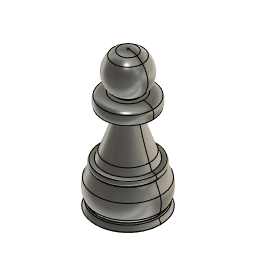
Pawn v1 (Autodesk Fusion 360 design; units mm, degrees)
Autodesk Fusion 360 part; units mm, degrees
sketch "pawn - side view" plane through (0, 0, 0) normal (0, 1, 0) x (1, 0, 0)
  spline S0 degree 3 poles (22.3033, -83.3947) (18.8902, -82.2834) (16.0063, -79.2936) (15.0802, -75.854) knots 0 0 0 0 1 1 1 1
  spline S1 degree 3 poles (15.0802, -75.854) (14.604, -74.0813) (14.7098, -71.1709) (15.3183, -69.3982) knots 0 0 0 0 1 1 1 1
  spline S2 degree 3 poles (15.3183, -69.3982) (15.9533, -67.5726) (16.5619, -66.6201) (18.361, -64.7944) knots 0 0 0 0 1 1 1 1
  line L0 (18.361, -64.7944) -> (19.684, -63.3922)
  line L1 (19.684, -63.3922) -> (17.1969, -63.3922)
  spline S3 degree 3 poles (17.1969, -63.3922) (15.239, -63.3922) (14.4981, -63.2863) (13.5985, -62.8365) knots 0 0 0 0 1 1 1 1
  spline S4 degree 3 poles (13.5985, -62.8365) (10.5558, -61.3813) (10.4235, -57.0686) (13.3604, -55.3753) knots 0 0 0 0 1 1 1 1
  spline S5 degree 3 poles (13.3604, -55.3753) (13.6515, -55.1901) (15.2125, -55.0049) (16.8, -54.9255) knots 0 0 0 0 1 1 1 1
  line L2 (16.8, -54.9255) -> (19.7104, -54.7932)
  line L3 (19.7104, -54.7932) -> (19.7898, -53.973)
  spline S6 degree 3 poles (19.7898, -53.973) (19.9485, -52.4384) (16.0592, -38.8124) (13.969, -33.5207) knots 0 0 0 0 1 1 1 1
  spline S7 degree 3 poles (13.969, -33.5207) (13.5456, -32.4359) (13.2546, -31.404) (13.334, -31.1924) knots 0 0 0 0 1 1 1 1
  spline S8 degree 3 poles (13.334, -31.1924) (13.5456, -30.6897) (38.3106, -30.6632) (38.5223, -31.1924) knots 0 0 0 0 1 1 1 1
  spline S9 degree 3 poles (38.5223, -31.1924) (38.6017, -31.404) (37.9667, -33.2032) (37.1465, -35.2405) knots 0 0 0 0 1 1 1 1
  spline S10 degree 3 poles (37.1465, -35.2405) (34.236, -42.3842) (30.8758, -53.3909) (31.2992, -54.4757) knots 0 0 0 0 1 1 1 1
  spline S11 degree 3 poles (31.2992, -54.4757) (31.4315, -54.8461) (31.8548, -54.9255) (34.0244, -54.9255) knots 0 0 0 0 1 1 1 1
  spline S12 degree 3 poles (34.0244, -54.9255) (36.9348, -54.9255) (38.0196, -55.2959) (38.9721, -56.6188) knots 0 0 0 0 1 1 1 1
  spline S13 degree 3 poles (38.9721, -56.6188) (39.7658, -57.7565) (39.7923, -60.3759) (38.9985, -61.4607) knots 0 0 0 0 1 1 1 1
  spline S14 degree 3 poles (38.9985, -61.4607) (38.0196, -62.8101) (36.4321, -63.3922) (33.8392, -63.3922) knots 0 0 0 0 1 1 1 1
  line L4 (33.8392, -63.3922) -> (31.5108, -63.3922)
  line L5 (31.5108, -63.3922) -> (32.966, -64.8474)
  spline S15 degree 3 poles (32.966, -64.8474) (37.3317, -69.213) (37.4904, -76.0392) (33.31, -80.4578) knots 0 0 0 0 1 1 1 1
  spline S16 degree 3 poles (33.31, -80.4578) (32.4104, -81.4103) (31.2992, -82.2305) (30.1879, -82.7597) knots 0 0 0 0 1 1 1 1
  spline S17 degree 3 poles (30.1879, -82.7597) (28.6533, -83.5005) (28.1242, -83.6063) (25.9281, -83.6857) knots 0 0 0 0 1 1 1 1
  spline S18 degree 3 poles (25.9281, -83.6857) (24.3142, -83.7386) (23.0177, -83.6328) (22.3033, -83.3947) knots 0 0 0 0 1 1 1 1
  spline S19 degree 3 poles (11.1115, -29.7901) (10.5294, -29.208) (10.3971, -27.6999) (10.8998, -27.1972) knots 0 0 0 0 1 1 1 1
  spline S20 degree 3 poles (10.8998, -27.1972) (11.1379, -26.959) (14.8156, -26.8797) (25.7958, -26.8797) knots 0 0 0 0 1 1 1 1
  spline S21 degree 3 poles (25.7958, -26.8797) (39.6071, -26.8797) (40.4273, -26.9061) (40.8242, -27.3559) knots 0 0 0 0 1 1 1 1
  spline S22 degree 3 poles (40.8242, -27.3559) (41.4856, -28.0967) (41.3798, -29.1286) (40.586, -29.7636) knots 0 0 0 0 1 1 1 1
  spline S23 degree 3 poles (40.586, -29.7636) (39.8981, -30.3192) (39.6335, -30.3192) (25.7694, -30.3192) knots 0 0 0 0 1 1 1 1
  spline S24 degree 3 poles (25.7694, -30.3192) (11.9846, -30.3192) (11.6406, -30.3192) (11.1115, -29.7901) knots 0 0 0 0 1 1 1 1
  spline S25 degree 3 poles (10.0267, -24.3132) (8.1746, -21.4028) (7.3015, -18.4924) (7.4867, -15.8201) knots 0 0 0 0 1 1 1 1
  spline S26 degree 3 poles (7.4867, -15.8201) (7.6454, -13.5182) (8.4921, -10.9517) (9.4181, -10.0257) knots 0 0 0 0 1 1 1 1
  line L6 (9.4181, -10.0257) -> (10.0267, -9.4172)
  line L7 (10.0267, -9.4172) -> (25.5313, -9.4172)
  spline S27 degree 3 poles (25.5313, -9.4172) (34.8181, -9.4172) (41.221, -9.523) (41.5121, -9.6817) knots 0 0 0 0 1 1 1 1
  spline S28 degree 3 poles (41.5121, -9.6817) (41.7767, -9.814) (42.3323, -10.6607) (42.7292, -11.5867) knots 0 0 0 0 1 1 1 1
  spline S29 degree 3 poles (42.7292, -11.5867) (43.814, -13.9415) (43.9727, -17.3017) (43.126, -20.0534) knots 0 0 0 0 1 1 1 1
  spline S30 degree 3 poles (43.126, -20.0534) (42.4381, -22.3024) (41.221, -24.8953) (40.4273, -25.7684) knots 0 0 0 0 1 1 1 1
  line L8 (40.4273, -25.7684) -> (39.8717, -26.3505)
  line L9 (39.8717, -26.3505) -> (25.6106, -26.3505)
  line L10 (25.6106, -26.3505) -> (11.3496, -26.3505)
  line L11 (11.3496, -26.3505) -> (10.0267, -24.3132)
  spline S31 degree 3 poles (8.8096, -8.4911) (8.1481, -8.0413) (7.7777, -6.6126) (8.0423, -5.5807) knots 0 0 0 0 1 1 1 1
  line L12 (8.0423, -5.5807) -> (8.201, -4.9192)
  line L13 (8.201, -4.9192) -> (25.3725, -4.9192)
  spline S32 degree 3 poles (25.3725, -4.9192) (40.639, -4.9192) (42.5969, -4.9722) (42.9673, -5.3426) knots 0 0 0 0 1 1 1 1
  spline S33 degree 3 poles (42.9673, -5.3426) (43.2054, -5.5542) (43.3906, -5.7924) (43.3906, -5.8188) knots 0 0 0 0 1 1 1 1
  spline S34 degree 3 poles (43.3906, -5.8188) (43.3906, -6.2686) (42.6763, -7.8297) (42.2529, -8.3059) knots 0 0 0 0 1 1 1 1
  line L14 (42.2529, -8.3059) -> (41.7238, -8.888)
  line L15 (41.7238, -8.888) -> (25.5313, -8.888)
  spline S35 degree 3 poles (25.5313, -8.888) (11.4554, -8.888) (9.3123, -8.8351) (8.8096, -8.4911) knots 0 0 0 0 1 1 1 1
  line L16 (25.3725, -4.9192) -> (25.3725, -83.6978)
  dimension "d1" = 78.7786
  constraint coincident S18 L16.end
  constraint perpendicular L13 L16
  measures "d1" distance of L13.end L16.end
revolve "Revolve1" add sketch "pawn - side view" angle 360 about axis through (25.3725, 0, 4.9192) along (0, 0, 1) contours S8 S9 S10 S11 S12 S13 S14 L4 L5 S15 S16 S17 S18 L16 makes body 1
revolve "Revolve2" add sketch "pawn - side view" angle 360 about axis through (25.3725, 0, 4.9192) along (0, 0, 1) separate body contours S20 S21 S22 S23 S24 L16 | L7 S27 S28 S29 S30 L8 L9 L10 L16 | S32 S33 S34 L14 L15 S35 L16 makes body 2 at (36.2898, -5.1337, 26.9265) makes body 3 at (43.3395, -2.7081, 18.1465) makes body 4 at (15.1481, -9.2524, 4.9791)
move_body "Align1" bodies 1 to x (1, 0, 0) y (0, 1, 0) z (0, 0, 1) at (0, 0, -1.4288)
move_body "Align2" bodies 3 to x (1, 0, 0) y (0, 1, 0) z (0, 0, 1) at (0, 0, -0.7938)
move_body "Align3" bodies 2 to x (1, 0, 0) y (0, 1, 0) z (0, 0, 1) at (0, 0, -1.7992)
move_body "Align4" bodies 1 to x (1, 0, 0) y (0, 1, 0) z (0, 0, 1) at (0, 0, -1.7992)
combine "Combine1" operation add target body 1 tool bodies 2 3 4
named bodies: "pawn body", "pawn divider part", "pawn bottom part", "pawn base part"
